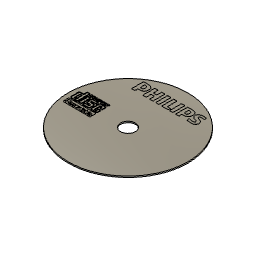
PhillipsCD (Autodesk Fusion 360 design; units mm, degrees)
Autodesk Fusion 360 part; units mm, degrees
(part 1 of 2)
sketch "Sketch1" plane through (0, 0, 0) normal (0, 0, 1) x (1, 0, 0)
  circle A0 centre (0, 0) radius 60
  circle A1 centre (0, 0) radius 7.5
  dimension "d1" = 120
  dimension "d2" = 15
  constraint coincident A0.centre A1.centre
  measures "d1" diameter of A0
  measures "d2" diameter of A1
extrude "Extrude1" add sketch "Sketch1" along normal blind 1.2 makes body 1
sketch "Sketch2" plane through (0, 0, 1.2) normal (0, 0, 1) x (-1, 0, 0)
  circle A0 centre (0, 0) radius 7.5
  circle A1 centre (0, 0) radius 60
  line L0 (-17.284, -38.4124) -> (-15.7727, -38.4124)
  line L1 (-15.7727, -38.4124) -> (-15.7527, -35.3898)
  line L2 (-15.7527, -35.3898) -> (-12.3726, -35.3898)
  line L3 (-12.3726, -35.3898) -> (-12.3726, -47.4806)
  spline S0 degree 3 poles (-12.3726, -47.4806) (-12.3738, -47.4644) (-15.1538, -47.4806) (-16.5283, -47.4806) knots 0 0 0 0 1 1 1 1
  spline S1 degree 3 poles (-16.5283, -47.4806) (-20.0822, -47.4806) (-22.1957, -46.2202) (-22.1957, -42.9463) knots 0 0 0 0 1 1 1 1
  spline S2 degree 3 poles (-22.1957, -42.9463) (-22.1957, -39.9661) (-20.5061, -38.4124) (-17.284, -38.4124) knots 0 0 0 0 1 1 1 1
  spline S3 degree 3 poles (-16.5283, -45.2133) (-16.3508, -45.2133) (-15.9744, -45.2258) (-15.7727, -45.2133) knots 0 0 0 0 1 1 1 1
  line L4 (-15.7727, -45.2133) -> (-15.7727, -40.6798)
  line L5 (-15.7727, -40.6798) -> (-16.5283, -40.6798)
  spline S4 degree 3 poles (-16.5283, -40.6798) (-18.3283, -40.6798) (-18.8516, -41.3599) (-18.8516, -42.8746) knots 0 0 0 0 1 1 1 1
  spline S5 degree 3 poles (-18.8516, -42.8746) (-18.8516, -44.3405) (-18.2346, -45.2133) (-16.5283, -45.2133) knots 0 0 0 0 1 1 1 1
  line L6 (13.6977, -35.3898) -> (13.6977, -40.3019)
  line L7 (13.6977, -40.3019) -> (17.0985, -40.3019)
  line L8 (17.0985, -40.3019) -> (17.0985, -35.3898)
  line L9 (17.0985, -35.3898) -> (20.4985, -35.3898)
  line L10 (20.4985, -35.3898) -> (20.4985, -47.4806)
  line L11 (20.4985, -47.4806) -> (17.0985, -47.4806)
  line L12 (17.0985, -47.4806) -> (17.0985, -42.5685)
  line L13 (17.0985, -42.5685) -> (13.6977, -42.5685)
  line L14 (13.6977, -42.5685) -> (13.6977, -47.4806)
  line L15 (13.6977, -47.4806) -> (10.2969, -47.4806)
  line L16 (10.2969, -47.4806) -> (10.2969, -35.3898)
  line L17 (10.2969, -35.3898) -> (13.6977, -35.3898)
  line L18 (7.6525, -35.3898) -> (7.6525, -47.4806)
  line L19 (7.6525, -47.4806) -> (4.2524, -47.4806)
  line L20 (4.2524, -47.4806) -> (4.2524, -35.3898)
  line L21 (4.2524, -35.3898) -> (7.6525, -35.3898)
  line L22 (-4.7889, -35.3898) -> (1.6076, -35.3898)
  line L23 (1.6076, -35.3898) -> (1.6076, -47.4806)
  line L24 (1.6076, -47.4806) -> (-1.7932, -47.4806)
  line L25 (-1.7932, -47.4806) -> (-1.7932, -37.6572)
  line L26 (-1.7932, -37.6572) -> (-5.1936, -37.6572)
  line L27 (-5.1936, -37.6572) -> (-4.7889, -35.3898)
  line L28 (-6.3271, -35.3898) -> (-6.3271, -47.4806)
  line L29 (-6.3271, -47.4806) -> (-9.7271, -47.4806)
  line L30 (-9.7271, -47.4806) -> (-9.7271, -35.3898)
  line L31 (-9.7271, -35.3898) -> (-6.3271, -35.3898)
  line L32 (-26.73, -44.458) -> (-26.73, -44.0798)
  spline S6 degree 3 poles (-26.73, -44.0798) (-26.73, -42.2239) (-32.3966, -43.0763) (-32.3966, -39.1685) knots 0 0 0 0 1 1 1 1
  spline S7 degree 3 poles (-32.3966, -39.1685) (-32.3966, -36.2373) (-30.3749, -35.3898) (-27.4853, -35.3898) knots 0 0 0 0 1 1 1 1
  spline S8 degree 3 poles (-27.4853, -35.3898) (-26.348, -35.3898) (-24.5129, -35.601) (-23.3292, -35.7677) knots 0 0 0 0 1 1 1 1
  line L33 (-23.3292, -35.7677) -> (-23.3292, -38.4124)
  spline S9 degree 3 poles (-23.3292, -38.4124) (-24.3724, -37.8759) (-26.348, -37.6572) (-27.4853, -37.6572) knots 0 0 0 0 1 1 1 1
  spline S10 degree 3 poles (-27.4853, -37.6572) (-28.7646, -37.6572) (-28.9966, -38.058) (-28.9966, -38.7906) knots 0 0 0 0 1 1 1 1
  spline S11 degree 3 poles (-28.9966, -38.7906) (-28.9966, -40.8725) (-23.3292, -39.9774) (-23.3292, -44.0798) knots 0 0 0 0 1 1 1 1
  spline S12 degree 3 poles (-23.3292, -44.0798) (-23.3292, -46.4616) (-25.6581, -47.4806) (-28.4532, -47.4806) knots 0 0 0 0 1 1 1 1
  spline S13 degree 3 poles (-28.4532, -47.4806) (-30.4338, -47.4806) (-30.741, -47.2978) (-31.6413, -47.1024) knots 0 0 0 0 1 1 1 1
  line L34 (-31.6413, -47.1024) -> (-31.6413, -44.8358)
  spline S14 degree 3 poles (-31.6413, -44.8358) (-30.8351, -45.177) (-29.7091, -45.2133) (-28.6187, -45.2133) knots 0 0 0 0 1 1 1 1
  spline S15 degree 3 poles (-28.6187, -45.2133) (-27.6243, -45.2133) (-26.73, -45.0931) (-26.73, -44.458) knots 0 0 0 0 1 1 1 1
  line L35 (26.9215, -38.4124) -> (28.4332, -38.4124)
  line L36 (28.4332, -38.4124) -> (28.4529, -35.3898)
  line L37 (28.4529, -35.3898) -> (31.8333, -35.3898)
  line L38 (31.8333, -35.3898) -> (31.8333, -47.4806)
  spline S16 degree 3 poles (31.8333, -47.4806) (31.8318, -47.4644) (29.0517, -47.4806) (27.6772, -47.4806) knots 0 0 0 0 1 1 1 1
  spline S17 degree 3 poles (27.6772, -47.4806) (24.1234, -47.4806) (22.0098, -46.2202) (22.0098, -42.9463) knots 0 0 0 0 1 1 1 1
  spline S18 degree 3 poles (22.0098, -42.9463) (22.0098, -39.9661) (23.6995, -38.4124) (26.9215, -38.4124) knots 0 0 0 0 1 1 1 1
  spline S19 degree 3 poles (27.6772, -45.2133) (27.8548, -45.2133) (28.2311, -45.2258) (28.4332, -45.2133) knots 0 0 0 0 1 1 1 1
  line L39 (28.4332, -45.2133) -> (28.4332, -40.6798)
  line L40 (28.4332, -40.6798) -> (27.6772, -40.6798)
  spline S20 degree 3 poles (27.6772, -40.6798) (25.8772, -40.6798) (25.3539, -41.3599) (25.3539, -42.8746) knots 0 0 0 0 1 1 1 1
  spline S21 degree 3 poles (25.3539, -42.8746) (25.3539, -44.3405) (25.9713, -45.2133) (27.6772, -45.2133) knots 0 0 0 0 1 1 1 1
extrude "Extrude2" add sketch "Sketch2" along normal blind 0.0254 separate body contours L0 L1 L2 L3 S0 S1 S2 | L6 L7 L8 L9 L10 L11 L12 L13 L14 L15 L16 L17 | L18 L19 L20 L21 | L22 L23 L24 L25 L26 L27 | L28 L29 L30 L31 | L32 S6 S7 S8 L33 S9 S10 S11 S12 S13 L34 S14 S15 | L35 L36 L37 L38 S16 S17 S18 makes body 2 at (-6.5191, 43.4504, 1.2) makes body 3 at (27.2121, 41.2566, 1.2) makes body 4 at (-0.474, 40.1759, 1.2) makes body 5 at (-11.4305, 41.0575, 1.2) makes body 6 at (13.506, 41.1834, 1.2) makes body 7 at (8.5938, 39.4201, 1.2) makes body 8 at (-30.6999, 41.1834, 1.2)
sketch "Sketch3" plane through (0, 0, 1.2) normal (0, 0, 1) x (-1, 0, 0)
  circle A0 centre (0, 0) radius 7.5
  circle A1 centre (0, 0) radius 60
  spline S0 degree 3 poles (28.7629, 10.1095) (28.3447, 10.1095) (28.0048, 9.7734) (28.0048, 9.3591) knots 0 0 0 0 1 1 1 1
  line L0 (28.0048, 9.3591) -> (28.0048, 4.8183)
  spline S1 degree 3 poles (28.0048, 4.8183) (28.0071, 4.4016) (28.3462, 4.0655) (28.7629, 4.0671) knots 0 0 0 0 1 1 1 1
  line L1 (28.7629, 4.0671) -> (54.5592, 4.0671)
  spline S2 degree 3 poles (54.5592, 4.0671) (54.9759, 4.0648) (55.315, 4.4008) (55.3173, 4.8175) knots 0 0 0 0 1 1 1 1
  line L2 (55.3173, 4.8175) -> (55.3173, 9.3591)
  spline S3 degree 3 poles (55.3173, 9.3591) (55.3173, 9.7734) (54.9789, 10.1095) (54.5592, 10.1095) knots 0 0 0 0 1 1 1 1
  line L3 (54.5592, 10.1095) -> (28.7629, 10.1095)
  spline S4 degree 3 poles (51.7003, -5.31) (52.3594, -5.31) (52.9732, -4.9141) (52.9732, -4.0332) knots 0 0 0 0 1 1 1 1
  spline S5 degree 3 poles (52.9732, -4.0332) (52.9732, -0.3901) (52.9671, -0.1162) (52.9671, 0.5345) knots 0 0 0 0 1 1 1 1
  spline S6 degree 3 poles (52.9671, 0.5345) (52.9671, 0.7869) (52.8021, 1.1521) (52.5819, 1.3386) knots 0 0 0 0 1 1 1 1
  spline S7 degree 3 poles (52.5819, 1.3386) (52.3602, 1.5235) (52.1407, 1.6524) (51.7678, 1.6524) knots 0 0 0 0 1 1 1 1
  spline S8 degree 3 poles (51.7678, 1.6524) (51.3619, 1.6524) (51.134, 1.5312) (50.8808, 1.2972) knots 0 0 0 0 1 1 1 1
  spline S9 degree 3 poles (50.8808, 1.2972) (50.6384, 1.0716) (50.5256, 0.767) (50.5256, 0.4063) knots 0 0 0 0 1 1 1 1
  spline S10 degree 3 poles (50.5256, 0.4063) (50.5256, 0.1646) (50.5355, -3.0357) (50.5355, -4.09) knots 0 0 0 0 1 1 1 1
  spline S11 degree 3 poles (50.5355, -4.09) (50.5355, -4.6402) (50.9744, -5.31) (51.7003, -5.31) knots 0 0 0 0 1 1 1 1
  line L4 (51.1195, -4.0332) -> (51.1195, 0.3802)
  spline S12 degree 3 poles (51.1195, 0.3802) (51.1195, 0.7915) (51.3504, 1.07) (51.7724, 1.07) knots 0 0 0 0 1 1 1 1
  spline S13 degree 3 poles (51.7724, 1.07) (52.1553, 1.0693) (52.3801, 0.7248) (52.3801, 0.4577) knots 0 0 0 0 1 1 1 1
  spline S14 degree 3 poles (52.3801, 0.4577) (52.3801, 0.3764) (52.3901, -2.0076) (52.3901, -4.1) knots 0 0 0 0 1 1 1 1
  spline S15 degree 3 poles (52.3901, -4.1) (52.3901, -4.4744) (52.0809, -4.723) (51.731, -4.723) knots 0 0 0 0 1 1 1 1
  spline S16 degree 3 poles (51.731, -4.723) (51.3811, -4.723) (51.1187, -4.4153) (51.1195, -4.0332) knots 0 0 0 0 1 1 1 1
  spline S17 degree 3 poles (41.3656, -7.4914) (41.1424, -7.4914) (40.8876, -7.4952) (40.6659, -7.4952) knots 0 0 0 0 1 1 1 1
  spline S18 degree 3 poles (40.6659, -7.4952) (40.6659, -8.1283) (40.6697, -9.2708) (40.6659, -9.4457) knots 0 0 0 0 1 1 1 1
  spline S19 degree 3 poles (40.6659, -9.4457) (40.5508, -9.0904) (40.2769, -8.3139) (39.9853, -7.4914) knots 0 0 0 0 1 1 1 1
  spline S20 degree 3 poles (39.9853, -7.4914) (39.7605, -7.4914) (39.5525, -7.4952) (39.3262, -7.4952) knots 0 0 0 0 1 1 1 1
  spline S21 degree 3 poles (39.3262, -7.4952) (39.109, -8.1451) (38.8842, -8.792) (38.6517, -9.4357) knots 0 0 0 0 1 1 1 1
  line L5 (38.6517, -9.4357) -> (38.6517, -7.4952)
  spline S22 degree 3 poles (38.6517, -7.4952) (38.4269, -7.4914) (38.2021, -7.4914) (37.9773, -7.4952) knots 0 0 0 0 1 1 1 1
  line L6 (37.9773, -7.4952) -> (37.975, -10.2061)
  spline S23 degree 3 poles (37.975, -10.2061) (38.3034, -10.2061) (38.6494, -10.2099) (38.9824, -10.2061) knots 0 0 0 0 1 1 1 1
  spline S24 degree 3 poles (38.9824, -10.2061) (39.3346, -9.1442) (39.5019, -8.6684) (39.6615, -8.2357) knots 0 0 0 0 1 1 1 1
  spline S25 degree 3 poles (39.6615, -8.2357) (39.7582, -8.5296) (40.0267, -9.2807) (40.3551, -10.2061) knots 0 0 0 0 1 1 1 1
  line L7 (40.3551, -10.2061) -> (41.3664, -10.2061)
  spline S26 degree 3 poles (41.3664, -10.2061) (41.3702, -9.9513) (41.3641, -8.3139) (41.3656, -7.4914) knots 0 0 0 0 1 1 1 1
  spline S27 degree 3 poles (27.9756, -0.4945) (27.9756, -0.9272) (28.2281, -1.2042) (28.5319, -1.1942) knots 0 0 0 0 1 1 1 1
  spline S28 degree 3 poles (28.5319, -1.1942) (29.0644, -1.1774) (29.9353, -1.2065) (30.5123, -1.1981) knots 0 0 0 0 1 1 1 1
  spline S29 degree 3 poles (30.5123, -1.1981) (30.9405, -1.1935) (31.0156, -0.8006) (31.0156, -0.4108) knots 0 0 0 0 1 1 1 1
  spline S30 degree 3 poles (31.0156, -0.4108) (31.0156, 0.1646) (30.985, 0.2483) (30.985, 0.4539) knots 0 0 0 0 1 1 1 1
  spline S31 degree 3 poles (30.985, 0.4539) (30.985, 0.691) (31.0885, 1.103) (31.4783, 1.103) knots 0 0 0 0 1 1 1 1
  spline S32 degree 3 poles (31.4783, 1.103) (31.8681, 1.103) (32.0246, 0.8184) (32.0246, 0.3818) knots 0 0 0 0 1 1 1 1
  spline S33 degree 3 poles (32.0246, 0.3818) (32.0246, 0.1071) (32.0246, -3.7723) (32.0346, -4.0885) knots 0 0 0 0 1 1 1 1
  spline S34 degree 3 poles (32.0346, -4.0885) (32.0446, -4.3309) (31.8712, -4.6885) (31.5121, -4.6839) knots 0 0 0 0 1 1 1 1
  spline S35 degree 3 poles (31.5121, -4.6839) (31.2397, -4.6854) (31.0179, -4.4667) (31.0164, -4.1944) knots 0 0 0 0 1 1 1 1
  spline S36 degree 3 poles (31.0164, -4.1944) (31.0164, -4.1898) (31.0164, -4.1859) (31.0164, -4.1813) knots 0 0 0 0 1 1 1 1
  spline S37 degree 3 poles (31.0164, -4.1813) (31.0226, -3.7286) (31.0241, -3.5475) (31.0264, -3.0181) knots 0 0 0 0 1 1 1 1
  spline S38 degree 3 poles (31.0264, -3.0181) (31.0287, -2.6153) (30.7693, -2.3582) (30.3987, -2.3582) knots 0 0 0 0 1 1 1 1
  line L8 (30.3987, -2.3582) -> (28.6048, -2.3621)
  spline S39 degree 3 poles (28.6048, -2.3621) (28.1905, -2.3621) (27.9887, -2.6099) (27.9987, -3.0895) knots 0 0 0 0 1 1 1 1
  spline S40 degree 3 poles (27.9987, -3.0895) (28.0086, -3.5728) (28.0048, -3.9166) (28.0048, -5.1189) knots 0 0 0 0 1 1 1 1
  spline S41 degree 3 poles (28.0048, -5.1189) (28.0048, -5.7266) (28.456, -6.8208) (29.6974, -6.8208) knots 0 0 0 0 1 1 1 1
  spline S42 degree 3 poles (29.6974, -6.8208) (30.121, -6.8208) (32.6131, -6.8285) (33.4372, -6.8208) knots 0 0 0 0 1 1 1 1
  spline S43 degree 3 poles (33.4372, -6.8208) (34.1339, -6.8147) (34.6196, -6.3405) (34.8682, -5.8402) knots 0 0 0 0 1 1 1 1
  spline S44 degree 3 poles (34.8682, -5.8402) (35.0884, -5.3975) (35.0316, -5.1397) (35.0316, -4.9333) knots 0 0 0 0 1 1 1 1
  spline S45 degree 3 poles (35.0316, -4.9333) (35.0316, -3.6074) (35.0293, 1.1698) (35.0278, 1.413) knots 0 0 0 0 1 1 1 1
  spline S46 degree 3 poles (35.0278, 1.413) (35.0178, 2.4228) (34.1669, 3.0819) (33.2746, 3.0719) knots 0 0 0 0 1 1 1 1
  spline S47 degree 3 poles (33.2746, 3.0719) (32.1574, 3.0658) (29.9875, 3.0719) (29.547, 3.0719) knots 0 0 0 0 1 1 1 1
  spline S48 degree 3 poles (29.547, 3.0719) (28.6294, 3.0719) (27.9887, 2.1765) (27.9887, 1.535) knots 0 0 0 0 1 1 1 1
  spline S49 degree 3 poles (27.9887, 1.535) (27.991, 0.7716) (27.9764, -0.2152) (27.9756, -0.4945) knots 0 0 0 0 1 1 1 1
  spline S50 degree 3 poles (28.5626, 1.3179) (28.5626, 2.0859) (29.099, 2.5033) (29.501, 2.5033) knots 0 0 0 0 1 1 1 1
  line L9 (29.501, 2.5033) -> (33.3221, 2.5033)
  spline S51 degree 3 poles (33.3221, 2.5033) (34.1869, 2.5033) (34.4593, 1.7637) (34.4593, 1.3447) knots 0 0 0 0 1 1 1 1
  spline S52 degree 3 poles (34.4593, 1.3447) (34.4593, -0.1937) (34.4431, -4.5634) (34.4554, -5.109) knots 0 0 0 0 1 1 1 1
  spline S53 degree 3 poles (34.4554, -5.109) (34.4654, -5.6545) (33.9459, -6.2085) (33.4196, -6.2192) knots 0 0 0 0 1 1 1 1
  spline S54 degree 3 poles (33.4196, -6.2192) (32.894, -6.2292) (30.1486, -6.2192) (29.7473, -6.2085) knots 0 0 0 0 1 1 1 1
  spline S55 degree 3 poles (29.7473, -6.2085) (29.3453, -6.1985) (28.5833, -5.9637) (28.5749, -5.1297) knots 0 0 0 0 1 1 1 1
  spline S56 degree 3 poles (28.5749, -5.1297) (28.5672, -4.2089) (28.5826, -3.5821) (28.5826, -3.3473) knots 0 0 0 0 1 1 1 1
  spline S57 degree 3 poles (28.5826, -3.3473) (28.5826, -3.1125) (28.5826, -2.9253) (28.8818, -2.9352) knots 0 0 0 0 1 1 1 1
  spline S58 degree 3 poles (28.8818, -2.9352) (29.1504, -2.9444) (29.9483, -2.9444) (30.1279, -2.9452) knots 0 0 0 0 1 1 1 1
  spline S59 degree 3 poles (30.1279, -2.9452) (30.279, -2.9475) (30.4486, -2.9966) (30.4402, -3.2859) knots 0 0 0 0 1 1 1 1
  spline S60 degree 3 poles (30.4402, -3.2859) (30.4363, -3.4532) (30.3872, -3.6419) (30.4363, -4.1913) knots 0 0 0 0 1 1 1 1
  spline S61 degree 3 poles (30.4363, -4.1913) (30.4808, -4.7) (30.8054, -5.2808) (31.5075, -5.2632) knots 0 0 0 0 1 1 1 1
  spline S62 degree 3 poles (31.5075, -5.2632) (32.0599, -5.2494) (32.5594, -4.9171) (32.6093, -4.1199) knots 0 0 0 0 1 1 1 1
  spline S63 degree 3 poles (32.6093, -4.1199) (32.6293, -3.8176) (32.607, -0.8029) (32.617, 0.5513) knots 0 0 0 0 1 1 1 1
  spline S64 degree 3 poles (32.617, 0.5513) (32.6185, 1.1751) (32.1205, 1.6854) (31.4975, 1.6984) knots 0 0 0 0 1 1 1 1
  spline S65 degree 3 poles (31.4975, 1.6984) (31.0486, 1.6984) (30.6427, 1.3578) (30.4985, 1.0086) knots 0 0 0 0 1 1 1 1
  spline S66 degree 3 poles (30.4985, 1.0086) (30.3565, 0.6626) (30.4271, -0.2489) (30.4271, -0.2888) knots 0 0 0 0 1 1 1 1
  spline S67 degree 3 poles (30.4271, -0.2888) (30.4271, -0.5068) (30.3435, -0.608) (30.1478, -0.608) knots 0 0 0 0 1 1 1 1
  line L10 (30.1478, -0.608) -> (28.9954, -0.6119)
  spline S68 degree 3 poles (28.9954, -0.6119) (28.8749, -0.6119) (28.5526, -0.6556) (28.5526, -0.2367) knots 0 0 0 0 1 1 1 1
  spline S69 degree 3 poles (28.5526, -0.2367) (28.5526, 0.2391) (28.5649, 0.7984) (28.5626, 1.3179) knots 0 0 0 0 1 1 1 1
  spline S70 degree 3 poles (35.8342, -1.4927) (35.8158, -1.9354) (35.9716, -2.3674) (36.2685, -2.6966) knots 0 0 0 0 1 1 1 1
  spline S71 degree 3 poles (36.2685, -2.6966) (36.5877, -3.0473) (37.0404, -3.2452) (37.5146, -3.2429) knots 0 0 0 0 1 1 1 1
  line L11 (37.5146, -3.2429) -> (39.8625, -3.2429)
  spline S72 degree 3 poles (39.8625, -3.2429) (40.1295, -3.2429) (40.2239, -3.4485) (40.2239, -3.655) knots 0 0 0 0 1 1 1 1
  spline S73 degree 3 poles (40.2239, -3.655) (40.2239, -3.7992) (40.1173, -4.0056) (39.7904, -4.0056) knots 0 0 0 0 1 1 1 1
  line L12 (39.7904, -4.0056) -> (36.6921, -4.0056)
  spline S74 degree 3 poles (36.6921, -4.0056) (36.4197, -4.0179) (36.1979, -4.2289) (36.1718, -4.5005) knots 0 0 0 0 1 1 1 1
  spline S75 degree 3 poles (36.1718, -4.5005) (36.1542, -4.7721) (36.1757, -5.8908) (36.1757, -6.2307) knots 0 0 0 0 1 1 1 1
  spline S76 degree 3 poles (36.1757, -6.2307) (36.178, -6.5584) (36.3875, -6.8216) (36.9744, -6.8108) knots 0 0 0 0 1 1 1 1
  spline S77 degree 3 poles (36.9744, -6.8108) (37.3166, -6.8047) (39.9369, -6.8001) (41.305, -6.8108) knots 0 0 0 0 1 1 1 1
  spline S78 degree 3 poles (41.305, -6.8108) (42.179, -6.8216) (42.9969, -6.0773) (42.9969, -5.2064) knots 0 0 0 0 1 1 1 1
  spline S79 degree 3 poles (42.9969, -5.2064) (42.9992, -4.5534) (42.9931, -2.6989) (42.9931, -2.339) knots 0 0 0 0 1 1 1 1
  spline S80 degree 3 poles (42.9931, -2.339) (42.9931, -1.0623) (42.1575, -0.4546) (41.1907, -0.4546) knots 0 0 0 0 1 1 1 1
  line L13 (41.1907, -0.4546) -> (39.1205, -0.4546)
  spline S81 degree 3 poles (39.1205, -0.4546) (38.6579, -0.4546) (38.6049, -0.2267) (38.6049, -0.0625) knots 0 0 0 0 1 1 1 1
  spline S82 degree 3 poles (38.6049, -0.0625) (38.6049, 0.1017) (38.7584, 0.2981) (39.0047, 0.2981) knots 0 0 0 0 1 1 1 1
  line L14 (39.0047, 0.2981) -> (42.4859, 0.2981)
  spline S83 degree 3 poles (42.4859, 0.2981) (42.7544, 0.2989) (43.003, 0.569) (43.003, 0.8552) knots 0 0 0 0 1 1 1 1
  line L15 (43.003, 0.8552) -> (43.003, 2.4934)
  spline S84 degree 3 poles (43.003, 2.4934) (43.003, 2.9161) (42.5603, 3.0803) (42.3539, 3.0803) knots 0 0 0 0 1 1 1 1
  spline S85 degree 3 poles (42.3539, 3.0803) (42.1475, 3.0803) (38.0509, 3.0681) (37.2131, 3.078) knots 0 0 0 0 1 1 1 1
  spline S86 degree 3 poles (37.2131, 3.078) (36.7366, 3.0842) (36.3115, 2.6798) (36.1872, 2.5056) knots 0 0 0 0 1 1 1 1
  spline S87 degree 3 poles (36.1872, 2.5056) (36.0959, 2.3775) (35.8258, 2.0092) (35.8258, 1.4429) knots 0 0 0 0 1 1 1 1
  spline S88 degree 3 poles (35.8258, 1.4429) (35.8258, 0.2644) (35.8197, -1.9646) (35.8342, -1.4927) knots 0 0 0 0 1 1 1 1
  spline S89 degree 3 poles (36.4235, 1.3486) (36.4235, 2.2762) (37.2499, 2.488) (37.4678, 2.488) knots 0 0 0 0 1 1 1 1
  line L16 (37.4678, 2.488) -> (42.1383, 2.4818)
  spline S90 degree 3 poles (42.1383, 2.4818) (42.4176, 2.4818) (42.4069, 2.2862) (42.4069, 2.0491) knots 0 0 0 0 1 1 1 1
  spline S91 degree 3 poles (42.4069, 2.0491) (42.4069, 1.812) (42.4145, 1.5573) (42.4107, 1.1636) knots 0 0 0 0 1 1 1 1
  spline S92 degree 3 poles (42.4107, 1.1636) (42.4107, 0.9465) (42.2534, 0.8751) (42.0662, 0.8751) knots 0 0 0 0 1 1 1 1
  line L17 (42.0662, 0.8751) -> (38.9563, 0.8751)
  spline S93 degree 3 poles (38.9563, 0.8751) (38.6379, 0.8751) (38.0203, 0.6066) (38.0287, -0.0939) knots 0 0 0 0 1 1 1 1
  spline S94 degree 3 poles (38.0287, -0.0939) (38.0348, -0.4431) (38.3379, -1.0416) (38.9563, -1.0416) knots 0 0 0 0 1 1 1 1
  line L18 (38.9563, -1.0416) -> (41.1815, -1.0416)
  spline S95 degree 3 poles (41.1815, -1.0416) (41.9296, -1.0416) (42.3969, -1.5042) (42.3969, -2.2355) knots 0 0 0 0 1 1 1 1
  spline S96 degree 3 poles (42.3969, -2.2355) (42.3969, -2.9667) (42.393, -4.5005) (42.393, -5.0783) knots 0 0 0 0 1 1 1 1
  spline S97 degree 3 poles (42.393, -5.0783) (42.393, -5.7128) (41.8974, -6.2116) (41.2636, -6.2116) knots 0 0 0 0 1 1 1 1
  line L19 (41.2636, -6.2116) -> (37.0304, -6.2116)
  spline S98 degree 3 poles (37.0304, -6.2116) (36.7389, -6.2108) (36.7427, -5.9768) (36.7427, -5.9116) knots 0 0 0 0 1 1 1 1
  line L20 (36.7427, -5.9116) -> (36.7427, -4.8504)
  spline S99 degree 3 poles (36.7427, -4.8504) (36.7427, -4.6448) (36.7834, -4.5857) (37.042, -4.5926) knots 0 0 0 0 1 1 1 1
  spline S100 degree 3 poles (37.042, -4.5926) (37.401, -4.6026) (39.5157, -4.5887) (39.8372, -4.5887) knots 0 0 0 0 1 1 1 1
  spline S101 degree 3 poles (39.8372, -4.5887) (40.5623, -4.5887) (40.8324, -3.9151) (40.8201, -3.645) knots 0 0 0 0 1 1 1 1
  spline S102 degree 3 poles (40.8201, -3.645) (40.8001, -3.1056) (40.418, -2.6521) (39.7904, -2.6429) knots 0 0 0 0 1 1 1 1
  spline S103 degree 3 poles (39.7904, -2.6429) (39.1627, -2.6321) (38.163, -2.6467) (37.6581, -2.646) knots 0 0 0 0 1 1 1 1
  spline S104 degree 3 poles (37.6581, -2.646) (36.7933, -2.646) (36.422, -2.2232) (36.422, -1.3469) knots 0 0 0 0 1 1 1 1
  line L21 (36.422, -1.3469) -> (36.4243, 1.3501)
  line L22 (36.4243, 1.3501) -> (36.4235, 1.3486)
  spline S105 degree 3 poles (35.1306, -9.4503) (35.1444, -9.6337) (35.1368, -9.8025) (35.2434, -9.946) knots 0 0 0 0 1 1 1 1
  spline S106 degree 3 poles (35.2434, -9.946) (35.3094, -10.0319) (35.3616, -10.1033) (35.5511, -10.1693) knots 0 0 0 0 1 1 1 1
  spline S107 degree 3 poles (35.5511, -10.1693) (35.8588, -10.279) (36.7849, -10.2061) (37.4072, -10.2061) knots 0 0 0 0 1 1 1 1
  spline S108 degree 3 poles (37.4072, -10.2061) (37.4049, -9.3552) (37.411, -7.7293) (37.411, -7.4952) knots 0 0 0 0 1 1 1 1
  spline S109 degree 3 poles (37.411, -7.4952) (37.1908, -7.4952) (36.956, -7.4914) (36.7366, -7.4914) knots 0 0 0 0 1 1 1 1
  spline S110 degree 3 poles (36.7366, -7.4914) (36.7366, -7.6863) (36.7427, -7.9633) (36.7366, -8.1275) knots 0 0 0 0 1 1 1 1
  spline S111 degree 3 poles (36.7366, -8.1275) (36.6391, -8.1206) (36.3207, -8.1229) (36.0775, -8.1283) knots 0 0 0 0 1 1 1 1
  spline S112 degree 3 poles (36.0775, -8.1283) (35.6792, -8.1375) (35.3102, -8.1827) (35.1966, -8.406) knots 0 0 0 0 1 1 1 1
  spline S113 degree 3 poles (35.1966, -8.406) (35.0953, -8.6101) (35.1091, -9.1779) (35.1306, -9.4503) knots 0 0 0 0 1 1 1 1
  spline S114 degree 3 poles (35.8611, -8.8472) (35.9486, -8.7175) (36.465, -8.7636) (36.7358, -8.7643) knots 0 0 0 0 1 1 1 1
  spline S115 degree 3 poles (36.7358, -8.7643) (36.7297, -9.003) (36.7419, -9.3452) (36.7358, -9.5784) knots 0 0 0 0 1 1 1 1
  spline S116 degree 3 poles (36.7358, -9.5784) (36.333, -9.5784) (36.0199, -9.6076) (35.8749, -9.5009) knots 0 0 0 0 1 1 1 1
  spline S117 degree 3 poles (35.8749, -9.5009) (35.7989, -9.4442) (35.7713, -8.9754) (35.8611, -8.8472) knots 0 0 0 0 1 1 1 1
  line L23 (34.2997, -8.0561) -> (33.4042, -8.0561)
  spline S118 degree 3 poles (33.4042, -8.0561) (33.3674, -7.928) (33.2676, -7.5712) (33.2393, -7.4945) knots 0 0 0 0 1 1 1 1
  line L24 (33.2393, -7.4945) -> (32.5648, -7.4945)
  spline S119 degree 3 poles (32.5648, -7.4945) (32.6262, -7.7262) (33.2646, -9.9068) (33.3766, -10.2061) knots 0 0 0 0 1 1 1 1
  spline S120 degree 3 poles (33.3766, -10.2061) (33.5922, -10.2015) (34.1109, -10.2099) (34.3426, -10.2061) knots 0 0 0 0 1 1 1 1
  spline S121 degree 3 poles (34.3426, -10.2061) (34.4746, -9.7833) (35.07, -7.7538) (35.1498, -7.4914) knots 0 0 0 0 1 1 1 1
  line L25 (35.1498, -7.4914) -> (34.4792, -7.4914)
  spline S122 degree 3 poles (34.4792, -7.4914) (34.4117, -7.7185) (34.3411, -7.9226) (34.3004, -8.0554) knots 0 0 0 0 1 1 1 1
  line L26 (34.3004, -8.0554) -> (34.2997, -8.0561)
  spline S123 degree 3 poles (33.8523, -9.5639) (33.751, -9.25) (33.6475, -8.8572) (33.5485, -8.4981) knots 0 0 0 0 1 1 1 1
  line L27 (33.5485, -8.4981) -> (34.1661, -8.4981)
  spline S124 degree 3 poles (34.1661, -8.4981) (34.0664, -8.8411) (33.9383, -9.26) (33.8523, -9.5639) knots 0 0 0 0 1 1 1 1
  spline S125 degree 3 poles (44.5, -6.8239) (44.8507, -6.8239) (45.8313, -6.8139) (46.4942, -6.8131) knots 0 0 0 0 1 1 1 1
  spline S126 degree 3 poles (46.4942, -6.8131) (46.9508, -6.8085) (47.0812, -6.4279) (47.0812, -6.1809) knots 0 0 0 0 1 1 1 1
  line L28 (47.0812, -6.1809) -> (47.0774, 2.3698)
  spline S127 degree 3 poles (47.0774, 2.3698) (47.0774, 2.8425) (46.8019, 3.0773) (46.4328, 3.0773) knots 0 0 0 0 1 1 1 1
  line L29 (46.4328, 3.0773) -> (44.3842, 3.0773)
  spline S128 degree 3 poles (44.3842, 3.0773) (44.0128, 3.0773) (43.8601, 2.6714) (43.8685, 2.3775) knots 0 0 0 0 1 1 1 1
  spline S129 degree 3 poles (43.8685, 2.3775) (43.8747, 2.1719) (43.8785, -2.6061) (43.8785, -6.088) knots 0 0 0 0 1 1 1 1
  spline S130 degree 3 poles (43.8785, -6.088) (43.8785, -6.6282) (44.1701, -6.8231) (44.5008, -6.8231) knots 0 0 0 0 1 1 1 1
  line L30 (44.5008, -6.8231) -> (44.5, -6.8239)
  spline S131 degree 3 poles (44.7241, 2.4811) (44.8369, 2.4811) (45.941, 2.4872) (46.2479, 2.4872) knots 0 0 0 0 1 1 1 1
  spline S132 degree 3 poles (46.2479, 2.4872) (46.4114, 2.4872) (46.5257, 2.409) (46.5257, 2.132) knots 0 0 0 0 1 1 1 1
  spline S133 degree 3 poles (46.5257, 2.132) (46.5257, 1.3908) (46.5134, -5.5095) (46.5134, -5.8601) knots 0 0 0 0 1 1 1 1
  spline S134 degree 3 poles (46.5134, -5.8601) (46.5172, -6.0819) (46.4605, -6.2116) (46.2157, -6.2116) knots 0 0 0 0 1 1 1 1
  line L31 (46.2157, -6.2116) -> (44.7341, -6.2116)
  spline S135 degree 3 poles (44.7341, -6.2116) (44.6113, -6.2116) (44.4525, -6.1341) (44.4525, -5.9077) knots 0 0 0 0 1 1 1 1
  spline S136 degree 3 poles (44.4525, -5.9077) (44.4525, 0.4447) (44.4448, 1.6378) (44.4448, 2.0806) knots 0 0 0 0 1 1 1 1
  spline S137 degree 3 poles (44.4448, 2.0806) (44.4448, 2.5233) (44.6098, 2.4818) (44.7241, 2.4811) knots 0 0 0 0 1 1 1 1
  spline S138 degree 3 poles (32.106, -7.5351) (31.6901, -7.3917) (30.7456, -7.4354) (30.4133, -7.542) knots 0 0 0 0 1 1 1 1
  spline S139 degree 3 poles (30.4133, -7.542) (30.2284, -7.6019) (30.1448, -7.7653) (30.1218, -7.9349) knots 0 0 0 0 1 1 1 1
  spline S140 degree 3 poles (30.1218, -7.9349) (30.0926, -8.1359) (30.0987, -8.2856) (30.0788, -8.4835) knots 0 0 0 0 1 1 1 1
  line L32 (30.0788, -8.4835) -> (30.7632, -8.4835)
  spline S141 degree 3 poles (30.7632, -8.4835) (30.7663, -8.396) (30.7778, -8.1989) (30.8246, -8.1428) knots 0 0 0 0 1 1 1 1
  spline S142 degree 3 poles (30.8246, -8.1428) (30.9305, -8.0193) (31.6786, -8.0362) (31.7561, -8.1636) knots 0 0 0 0 1 1 1 1
  spline S143 degree 3 poles (31.7561, -8.1636) (31.8374, -8.2948) (31.8006, -9.0283) (31.7891, -9.25) knots 0 0 0 0 1 1 1 1
  spline S144 degree 3 poles (31.7891, -9.25) (31.7768, -9.4503) (31.7499, -9.4802) (31.7154, -9.5439) knots 0 0 0 0 1 1 1 1
  spline S145 degree 3 poles (31.7154, -9.5439) (31.6563, -9.6521) (30.8407, -9.6306) (30.8062, -9.5178) knots 0 0 0 0 1 1 1 1
  spline S146 degree 3 poles (30.8062, -9.5178) (30.7693, -9.4043) (30.7693, -9.3367) (30.7693, -9.1825) knots 0 0 0 0 1 1 1 1
  line L33 (30.7693, -9.1825) -> (30.0734, -9.1825)
  spline S147 degree 3 poles (30.0734, -9.1825) (30.0734, -9.4365) (30.0865, -9.6621) (30.1041, -9.8002) knots 0 0 0 0 1 1 1 1
  spline S148 degree 3 poles (30.1041, -9.8002) (30.1248, -9.9721) (30.2921, -10.1186) (30.5453, -10.1762) knots 0 0 0 0 1 1 1 1
  spline S149 degree 3 poles (30.5453, -10.1762) (30.7709, -10.2268) (31.0202, -10.2437) (31.1814, -10.2375) knots 0 0 0 0 1 1 1 1
  spline S150 degree 3 poles (31.1814, -10.2375) (31.3563, -10.2314) (31.6425, -10.2306) (31.8919, -10.1999) knots 0 0 0 0 1 1 1 1
  spline S151 degree 3 poles (31.8919, -10.1999) (32.1328, -10.1693) (32.4359, -10.0802) (32.4612, -9.7818) knots 0 0 0 0 1 1 1 1
  spline S152 degree 3 poles (32.4612, -9.7818) (32.5211, -9.1656) (32.5234, -8.5449) (32.4674, -7.928) knots 0 0 0 0 1 1 1 1
  spline S153 degree 3 poles (32.4674, -7.928) (32.4382, -7.6357) (32.287, -7.5965) (32.106, -7.5336) knots 0 0 0 0 1 1 1 1
  line L34 (32.106, -7.5336) -> (32.106, -7.5351)
  line L35 (29.3015, -7.4937) -> (28.6179, -7.4937)
  line L36 (28.6179, -7.4937) -> (28.6179, -9.4772)
  line L37 (28.6179, -9.4772) -> (27.9833, -9.4772)
  line L38 (27.9833, -9.4772) -> (27.9833, -10.2053)
  line L39 (27.9833, -10.2053) -> (29.9192, -10.2053)
  line L40 (29.9192, -10.2053) -> (29.9192, -9.4718)
  line L41 (29.9192, -9.4718) -> (29.3015, -9.4718)
  line L42 (29.3015, -9.4718) -> (29.3015, -7.4937)
  spline S154 degree 3 poles (47.8861, -9.5792) (47.8861, -9.6398) (47.8861, -10.2069) (48.5038, -10.2069) knots 0 0 0 0 1 1 1 1
  spline S155 degree 3 poles (48.5038, -10.2069) (48.8851, -10.2069) (49.8987, -10.226) (50.6046, -10.2069) knots 0 0 0 0 1 1 1 1
  spline S156 degree 3 poles (50.6046, -10.2069) (50.9077, -10.1769) (51.134, -9.9145) (51.1195, -9.6099) knots 0 0 0 0 1 1 1 1
  spline S157 degree 3 poles (51.1195, -9.6099) (51.1056, -9.2577) (51.1195, -8.8081) (51.1195, -7.0656) knots 0 0 0 0 1 1 1 1
  spline S158 degree 3 poles (51.1195, -7.0656) (51.1172, -6.9136) (51.2261, -6.8231) (51.4133, -6.8231) knots 0 0 0 0 1 1 1 1
  spline S159 degree 3 poles (51.4133, -6.8231) (51.6005, -6.8231) (52.9993, -6.8269) (53.9109, -6.8193) knots 0 0 0 0 1 1 1 1
  spline S160 degree 3 poles (53.9109, -6.8193) (54.7871, -6.8139) (55.503, -5.9469) (55.503, -5.3307) knots 0 0 0 0 1 1 1 1
  spline S161 degree 3 poles (55.503, -5.3307) (55.4953, -2.1449) (55.5068, 0.4493) (55.5068, 1.3685) knots 0 0 0 0 1 1 1 1
  spline S162 degree 3 poles (55.5068, 1.3685) (55.5068, 2.2877) (54.8746, 2.7704) (54.4165, 2.9545) knots 0 0 0 0 1 1 1 1
  spline S163 degree 3 poles (54.4165, 2.9545) (54.1042, 3.0796) (53.66, 3.078) (53.2211, 3.078) knots 0 0 0 0 1 1 1 1
  spline S164 degree 3 poles (53.2211, 3.078) (52.6279, 3.078) (50.0276, 3.0719) (48.6634, 3.078) knots 0 0 0 0 1 1 1 1
  spline S165 degree 3 poles (48.6634, 3.078) (47.8331, 3.0819) (47.8823, 2.465) (47.8823, 2.2662) knots 0 0 0 0 1 1 1 1
  spline S166 degree 3 poles (47.8823, 2.2662) (47.8823, 2.132) (47.8861, -0.3541) (47.8861, -9.5792) knots 0 0 0 0 1 1 1 1
  spline S167 degree 3 poles (48.4876, 2.1366) (48.4876, 2.3737) (48.5552, 2.488) (48.816, 2.4872) knots 0 0 0 0 1 1 1 1
  spline S168 degree 3 poles (48.816, 2.4872) (51.4325, 2.4765) (53.4167, 2.4811) (53.808, 2.4811) knots 0 0 0 0 1 1 1 1
  spline S169 degree 3 poles (53.808, 2.4811) (54.2914, 2.4811) (54.9214, 2.0951) (54.9214, 1.3892) knots 0 0 0 0 1 1 1 1
  spline S170 degree 3 poles (54.9214, 1.3892) (54.9314, -2.0122) (54.9014, -4.8673) (54.9091, -5.2179) knots 0 0 0 0 1 1 1 1
  spline S171 degree 3 poles (54.9091, -5.2179) (54.9214, -5.6929) (54.4035, -6.2238) (53.8633, -6.2223) knots 0 0 0 0 1 1 1 1
  spline S172 degree 3 poles (53.8633, -6.2223) (53.0553, -6.22) (51.7156, -6.2215) (51.1816, -6.2223) knots 0 0 0 0 1 1 1 1
  spline S173 degree 3 poles (51.1816, -6.2223) (50.7795, -6.2223) (50.5309, -6.4195) (50.5386, -6.9067) knots 0 0 0 0 1 1 1 1
  spline S174 degree 3 poles (50.5386, -6.9067) (50.5248, -8.1566) (50.5225, -8.7559) (50.5325, -9.28) knots 0 0 0 0 1 1 1 1
  spline S175 degree 3 poles (50.5325, -9.28) (50.5401, -9.7027) (50.2532, -9.6084) (50.1672, -9.6206) knots 0 0 0 0 1 1 1 1
  spline S176 degree 3 poles (50.1672, -9.6206) (50.178, -9.6199) (49.126, -9.6268) (48.7654, -9.616) knots 0 0 0 0 1 1 1 1
  spline S177 degree 3 poles (48.7654, -9.616) (48.5084, -9.6206) (48.4969, -9.4281) (48.4938, -9.3436) knots 0 0 0 0 1 1 1 1
  spline S178 degree 3 poles (48.4938, -9.3436) (48.4861, -9.1871) (48.4876, 1.9417) (48.4876, 2.1366) knots 0 0 0 0 1 1 1 1
  spline S179 degree 3 poles (42.2204, -7.5106) (41.8122, -7.605) (41.8122, -7.8298) (41.7923, -7.974) knots 0 0 0 0 1 1 1 1
  spline S180 degree 3 poles (41.7923, -7.974) (41.7455, -8.3347) (41.7554, -9.4541) (41.8084, -9.8025) knots 0 0 0 0 1 1 1 1
  spline S181 degree 3 poles (41.8084, -9.8025) (41.8429, -10.0212) (41.9634, -10.0795) (42.1391, -10.1478) knots 0 0 0 0 1 1 1 1
  spline S182 degree 3 poles (42.1391, -10.1478) (42.4483, -10.2713) (43.2854, -10.2805) (43.7404, -10.1685) knots 0 0 0 0 1 1 1 1
  spline S183 degree 3 poles (43.7404, -10.1685) (44.0581, -10.091) (44.0987, -10.0166) (44.157, -9.8025) knots 0 0 0 0 1 1 1 1
  spline S184 degree 3 poles (44.157, -9.8025) (44.2284, -9.5516) (44.2062, -8.3646) (44.1778, -7.9901) knots 0 0 0 0 1 1 1 1
  spline S185 degree 3 poles (44.1778, -7.9901) (44.1532, -7.6518) (43.9307, -7.5689) (43.8256, -7.5367) knots 0 0 0 0 1 1 1 1
  spline S186 degree 3 poles (43.8256, -7.5367) (43.4849, -7.4293) (42.6792, -7.4062) (42.2204, -7.5106) knots 0 0 0 0 1 1 1 1
  spline S187 degree 3 poles (43.3491, -8.0976) (43.4228, -8.1252) (43.4573, -8.1682) (43.4696, -8.2372) knots 0 0 0 0 1 1 1 1
  spline S188 degree 3 poles (43.4696, -8.2372) (43.5041, -8.6308) (43.5102, -9.026) (43.4895, -9.4204) knots 0 0 0 0 1 1 1 1
  spline S189 degree 3 poles (43.4895, -9.4204) (43.4688, -9.5501) (43.4289, -9.5639) (43.3399, -9.5853) knots 0 0 0 0 1 1 1 1
  spline S190 degree 3 poles (43.3399, -9.5853) (43.1327, -9.6368) (42.7322, -9.6291) (42.6018, -9.5861) knots 0 0 0 0 1 1 1 1
  spline S191 degree 3 poles (42.6018, -9.5861) (42.5818, -9.5792) (42.5104, -9.5662) (42.4974, -9.4426) knots 0 0 0 0 1 1 1 1
  spline S192 degree 3 poles (42.4974, -9.4426) (42.4606, -9.1035) (42.4529, -8.4306) (42.4951, -8.2257) knots 0 0 0 0 1 1 1 1
  spline S193 degree 3 poles (42.4951, -8.2257) (42.5158, -8.1206) (42.5665, -8.0953) (42.6393, -8.0861) knots 0 0 0 0 1 1 1 1
  spline S194 degree 3 poles (42.6393, -8.0861) (42.8473, -8.063) (43.2125, -8.0431) (43.3491, -8.0976) knots 0 0 0 0 1 1 1 1
  spline S195 degree 3 poles (46.6208, -7.5451) (46.205, -7.4032) (45.2627, -7.4469) (44.9282, -7.552) knots 0 0 0 0 1 1 1 1
  spline S196 degree 3 poles (44.9282, -7.552) (44.7463, -7.6126) (44.6765, -7.6993) (44.6174, -7.9464) knots 0 0 0 0 1 1 1 1
  spline S197 degree 3 poles (44.6174, -7.9464) (44.5806, -8.1014) (44.5883, -8.2917) (44.5883, -8.4897) knots 0 0 0 0 1 1 1 1
  line L43 (44.5883, -8.4897) -> (45.2742, -8.4897)
  spline S198 degree 3 poles (45.2742, -8.4897) (45.2781, -8.403) (45.2934, -8.2104) (45.3417, -8.1551) knots 0 0 0 0 1 1 1 1
  spline S199 degree 3 poles (45.3417, -8.1551) (45.4453, -8.0316) (46.1957, -8.0477) (46.2732, -8.1751) knots 0 0 0 0 1 1 1 1
  spline S200 degree 3 poles (46.2732, -8.1751) (46.3546, -8.3063) (46.3362, -9.0091) (46.32, -9.2309) knots 0 0 0 0 1 1 1 1
  spline S201 degree 3 poles (46.32, -9.2309) (46.3139, -9.3137) (46.3162, -9.468) (46.2794, -9.5293) knots 0 0 0 0 1 1 1 1
  spline S202 degree 3 poles (46.2794, -9.5293) (46.1996, -9.659) (45.387, -9.6275) (45.321, -9.5293) knots 0 0 0 0 1 1 1 1
  spline S203 degree 3 poles (45.321, -9.5293) (45.2704, -9.4549) (45.2903, -9.339) (45.2742, -9.1902) knots 0 0 0 0 1 1 1 1
  spline S204 degree 3 poles (45.2742, -9.1902) (45.1093, -9.1856) (44.8162, -9.1902) (44.5883, -9.1902) knots 0 0 0 0 1 1 1 1
  spline S205 degree 3 poles (44.5883, -9.1902) (44.5883, -9.4442) (44.6028, -9.6751) (44.619, -9.8132) knots 0 0 0 0 1 1 1 1
  spline S206 degree 3 poles (44.619, -9.8132) (44.6397, -9.9851) (44.8069, -10.1317) (45.0602, -10.1884) knots 0 0 0 0 1 1 1 1
  spline S207 degree 3 poles (45.0602, -10.1884) (45.288, -10.2398) (45.5366, -10.256) (45.6962, -10.2498) knots 0 0 0 0 1 1 1 1
  spline S208 degree 3 poles (45.6962, -10.2498) (45.8727, -10.2452) (46.1589, -10.2429) (46.4067, -10.2107) knots 0 0 0 0 1 1 1 1
  spline S209 degree 3 poles (46.4067, -10.2107) (46.6477, -10.18) (46.9531, -10.091) (46.9776, -9.7917) knots 0 0 0 0 1 1 1 1
  spline S210 degree 3 poles (46.9776, -9.7917) (46.9976, -9.56) (47.0689, -8.7498) (46.9838, -7.938) knots 0 0 0 0 1 1 1 1
  spline S211 degree 3 poles (46.9838, -7.938) (46.9531, -7.6472) (46.8034, -7.6073) (46.6208, -7.5451) knots 0 0 0 0 1 1 1 1
  spline S212 degree 3 poles (46.9584, 6.6436) (46.7866, 6.5807) (46.5986, 6.573) (46.4221, 6.6206) knots 0 0 0 0 1 1 1 1
  spline S213 degree 3 poles (46.4221, 6.6206) (46.2241, 6.6805) (46.1014, 6.8086) (46.0346, 6.9966) knots 0 0 0 0 1 1 1 1
  spline S214 degree 3 poles (46.0346, 6.9966) (46.0147, 7.0534) (46.0139, 7.1071) (46.0016, 7.1677) knots 0 0 0 0 1 1 1 1
  spline S215 degree 3 poles (46.0016, 7.1677) (45.8689, 7.1715) (45.7223, 7.1715) (45.5673, 7.1677) knots 0 0 0 0 1 1 1 1
  spline S216 degree 3 poles (45.5673, 7.1677) (45.6003, 6.8654) (45.6978, 6.6037) (45.875, 6.4441) knots 0 0 0 0 1 1 1 1
  spline S217 degree 3 poles (45.875, 6.4441) (46.0515, 6.2861) (46.3139, 6.1771) (46.683, 6.1894) knots 0 0 0 0 1 1 1 1
  spline S218 degree 3 poles (46.683, 6.1894) (46.9638, 6.1978) (47.2339, 6.3022) (47.4472, 6.4848) knots 0 0 0 0 1 1 1 1
  spline S219 degree 3 poles (47.4472, 6.4848) (47.6513, 6.6636) (47.7733, 6.9436) (47.8347, 7.2697) knots 0 0 0 0 1 1 1 1
  spline S220 degree 3 poles (47.8347, 7.2697) (47.8753, 7.4808) (47.8861, 7.6964) (47.8677, 7.9104) knots 0 0 0 0 1 1 1 1
  spline S221 degree 3 poles (47.8677, 7.9104) (47.8063, 8.5097) (47.4694, 8.9447) (46.8886, 9.046) knots 0 0 0 0 1 1 1 1
  spline S222 degree 3 poles (46.8886, 9.046) (46.6784, 9.0829) (46.3914, 9.0621) (46.218, 8.9892) knots 0 0 0 0 1 1 1 1
  spline S223 degree 3 poles (46.218, 8.9892) (46.0269, 8.9041) (45.8673, 8.7606) (45.763, 8.5795) knots 0 0 0 0 1 1 1 1
  spline S224 degree 3 poles (45.763, 8.5795) (45.6655, 8.4284) (45.598, 8.2672) (45.5796, 8.0332) knots 0 0 0 0 1 1 1 1
  line L44 (45.5796, 8.0332) -> (46.0016, 8.0332)
  spline S225 degree 3 poles (46.0016, 8.0332) (46.0408, 8.1867) (46.0853, 8.3324) (46.1727, 8.4429) knots 0 0 0 0 1 1 1 1
  spline S226 degree 3 poles (46.1727, 8.4429) (46.4098, 8.7483) (46.9561, 8.7383) (47.1971, 8.4429) knots 0 0 0 0 1 1 1 1
  spline S227 degree 3 poles (47.1971, 8.4429) (47.3912, 8.202) (47.4556, 7.658) (47.3666, 7.2467) knots 0 0 0 0 1 1 1 1
  spline S228 degree 3 poles (47.3666, 7.2467) (47.3137, 6.992) (47.1702, 6.7396) (46.9584, 6.6436) knots 0 0 0 0 1 1 1 1
  spline S229 degree 3 poles (48.2659, 6.9413) (48.3296, 6.7549) (48.4477, 6.5585) (48.5843, 6.4411) knots 0 0 0 0 1 1 1 1
  spline S230 degree 3 poles (48.5843, 6.4411) (48.7746, 6.2776) (49.0938, 6.1403) (49.4851, 6.1902) knots 0 0 0 0 1 1 1 1
  spline S231 degree 3 poles (49.4851, 6.1902) (49.8266, 6.2331) (50.1197, 6.3866) (50.2931, 6.5999) knots 0 0 0 0 1 1 1 1
  spline S232 degree 3 poles (50.2931, 6.5999) (50.5969, 6.972) (50.6844, 7.5214) (50.5946, 7.9979) knots 0 0 0 0 1 1 1 1
  spline S233 degree 3 poles (50.5946, 7.9979) (50.4803, 8.6002) (50.122, 8.9731) (49.5588, 9.0261) knots 0 0 0 0 1 1 1 1
  spline S234 degree 3 poles (49.5588, 9.0261) (49.3171, 9.0468) (49.0355, 9.0468) (48.8352, 8.967) knots 0 0 0 0 1 1 1 1
  spline S235 degree 3 poles (48.8352, 8.967) (48.5214, 8.8427) (48.1853, 8.3915) (48.1976, 8.1368) knots 0 0 0 0 1 1 1 1
  line L45 (48.1976, 8.1368) -> (48.6319, 8.1368)
  spline S236 degree 3 poles (48.6319, 8.1368) (48.6503, 8.2304) (48.6887, 8.3194) (48.7447, 8.3977) knots 0 0 0 0 1 1 1 1
  spline S237 degree 3 poles (48.7447, 8.3977) (48.9365, 8.6424) (49.4161, 8.7598) (49.769, 8.581) knots 0 0 0 0 1 1 1 1
  spline S238 degree 3 poles (49.769, 8.581) (49.8995, 8.5143) (50.0299, 8.3432) (50.0782, 8.1936) knots 0 0 0 0 1 1 1 1
  spline S239 degree 3 poles (50.0782, 8.1936) (50.1189, 8.0662) (50.135, 7.9281) (50.135, 7.7608) knots 0 0 0 0 1 1 1 1
  line L46 (50.135, 7.7608) -> (48.1546, 7.7608)
  spline S240 degree 3 poles (48.1546, 7.7608) (48.1546, 7.4462) (48.1876, 7.1777) (48.2674, 6.9406) knots 0 0 0 0 1 1 1 1
  line L47 (48.2674, 6.9406) -> (48.2659, 6.9413)
  spline S241 degree 3 poles (50.1327, 7.3971) (50.1335, 7.2966) (50.1181, 7.1961) (50.0882, 7.1009) knots 0 0 0 0 1 1 1 1
  spline S242 degree 3 poles (50.0882, 7.1009) (50.023, 6.939) (49.9117, 6.8002) (49.7675, 6.702) knots 0 0 0 0 1 1 1 1
  spline S243 degree 3 poles (49.7675, 6.702) (49.6493, 6.6252) (49.512, 6.5823) (49.3716, 6.5777) knots 0 0 0 0 1 1 1 1
  spline S244 degree 3 poles (49.3716, 6.5777) (49.1897, 6.5754) (49.0132, 6.636) (48.8698, 6.748) knots 0 0 0 0 1 1 1 1
  spline S245 degree 3 poles (48.8698, 6.748) (48.7063, 6.8915) (48.6419, 7.1102) (48.6189, 7.3979) knots 0 0 0 0 1 1 1 1
  line L48 (48.6189, 7.3979) -> (50.1327, 7.3971)
  spline S246 degree 3 poles (30.8108, 8.558) (30.9067, 8.4744) (30.9804, 8.3693) (31.0264, 8.2503) knots 0 0 0 0 1 1 1 1
  spline S247 degree 3 poles (31.0264, 8.2503) (31.0732, 8.1184) (31.0832, 7.9734) (31.0832, 7.7946) knots 0 0 0 0 1 1 1 1
  line L49 (31.0832, 7.7946) -> (29.1128, 7.7946)
  spline S248 degree 3 poles (29.1128, 7.7946) (29.1204, 7.5107) (29.1304, 7.3695) (29.1718, 7.1915) knots 0 0 0 0 1 1 1 1
  spline S249 degree 3 poles (29.1718, 7.1915) (29.2294, 6.936) (29.3453, 6.7027) (29.4903, 6.5308) knots 0 0 0 0 1 1 1 1
  spline S250 degree 3 poles (29.4903, 6.5308) (29.6644, 6.3237) (30.0028, 6.1917) (30.411, 6.2247) knots 0 0 0 0 1 1 1 1
  spline S251 degree 3 poles (30.411, 6.2247) (31.1998, 6.2845) (31.5343, 6.9214) (31.575, 7.5851) knots 0 0 0 0 1 1 1 1
  spline S252 degree 3 poles (31.575, 7.5851) (31.6195, 8.2918) (31.2995, 9.0338) (30.4578, 9.0829) knots 0 0 0 0 1 1 1 1
  spline S253 degree 3 poles (30.4578, 9.0829) (30.2376, 9.0967) (29.9913, 9.0806) (29.8202, 9.0153) knots 0 0 0 0 1 1 1 1
  spline S254 degree 3 poles (29.8202, 9.0153) (29.4688, 8.8749) (29.2632, 8.5642) (29.1596, 8.1713) knots 0 0 0 0 1 1 1 1
  line L50 (29.1596, 8.1713) -> (29.6046, 8.1713)
  spline S255 degree 3 poles (29.6046, 8.1713) (29.6982, 8.6516) (30.3819, 8.891) (30.8115, 8.5588) knots 0 0 0 0 1 1 1 1
  line L51 (30.8115, 8.5588) -> (30.8108, 8.558)
  spline S256 degree 3 poles (31.0272, 7.1002) (30.9366, 6.8769) (30.7126, 6.6567) (30.434, 6.6206) knots 0 0 0 0 1 1 1 1
  spline S257 degree 3 poles (30.434, 6.6206) (30.0581, 6.5738) (29.8217, 6.7434) (29.7059, 6.9628) knots 0 0 0 0 1 1 1 1
  spline S258 degree 3 poles (29.7059, 6.9628) (29.6307, 7.1086) (29.5939, 7.2713) (29.5977, 7.4355) knots 0 0 0 0 1 1 1 1
  line L52 (29.5977, 7.4355) -> (31.0847, 7.4355)
  spline S259 degree 3 poles (31.0847, 7.4355) (31.087, 7.3212) (31.0671, 7.2076) (31.0272, 7.1002) knots 0 0 0 0 1 1 1 1
  spline S260 degree 3 poles (51.0335, 8.8312) (51.0972, 8.7967) (51.1049, 8.6002) (51.1133, 8.4215) knots 0 0 0 0 1 1 1 1
  spline S261 degree 3 poles (51.1133, 8.4215) (51.1371, 7.9411) (51.101, 7.414) (51.4087, 7.226) knots 0 0 0 0 1 1 1 1
  spline S262 degree 3 poles (51.4087, 7.226) (51.553, 7.1385) (51.6389, 7.1692) (51.4655, 7.0549) knots 0 0 0 0 1 1 1 1
  spline S263 degree 3 poles (51.4655, 7.0549) (51.2376, 6.9045) (51.1195, 6.6958) (51.078, 6.349) knots 0 0 0 0 1 1 1 1
  spline S264 degree 3 poles (51.078, 6.349) (51.0074, 5.7298) (51.3888, 5.3676) (51.886, 5.2794) knots 0 0 0 0 1 1 1 1
  spline S265 degree 3 poles (51.886, 5.2794) (52.1238, 5.2364) (53.2525, 5.2449) (54.026, 5.2449) knots 0 0 0 0 1 1 1 1
  line L53 (54.026, 5.2449) -> (54.026, 8.9678)
  spline S266 degree 3 poles (54.026, 8.9678) (53.8648, 8.9678) (53.6853, 8.9739) (53.5264, 8.9678) knots 0 0 0 0 1 1 1 1
  line L54 (53.5264, 8.9678) -> (53.5264, 7.3626)
  line L55 (53.5264, 7.3626) -> (52.199, 7.3626)
  spline S267 degree 3 poles (52.199, 7.3626) (52.0532, 7.3565) (51.9113, 7.4102) (51.8062, 7.5107) knots 0 0 0 0 1 1 1 1
  spline S268 degree 3 poles (51.8062, 7.5107) (51.6159, 7.6849) (51.6297, 8.067) (51.6182, 8.4383) knots 0 0 0 0 1 1 1 1
  spline S269 degree 3 poles (51.6182, 8.4383) (51.6113, 8.6163) (51.5875, 8.7944) (51.5468, 8.9678) knots 0 0 0 0 1 1 1 1
  line L56 (51.5468, 8.9678) -> (50.9307, 8.9678)
  spline S270 degree 3 poles (50.9307, 8.9678) (50.9583, 8.8665) (50.9261, 8.8903) (51.0335, 8.8312) knots 0 0 0 0 1 1 1 1
  spline S271 degree 3 poles (51.8185, 6.8278) (51.9527, 6.8984) (52.1024, 6.9337) (52.2543, 6.9314) knots 0 0 0 0 1 1 1 1
  spline S272 degree 3 poles (52.2543, 6.9314) (52.674, 6.9314) (53.2472, 6.9344) (53.5272, 6.9306) knots 0 0 0 0 1 1 1 1
  spline S273 degree 3 poles (53.5272, 6.9306) (53.5272, 6.5155) (53.5311, 6.049) (53.5311, 5.6738) knots 0 0 0 0 1 1 1 1
  spline S274 degree 3 poles (53.5311, 5.6738) (53.2395, 5.6738) (52.6072, 5.6692) (52.2282, 5.6692) knots 0 0 0 0 1 1 1 1
  spline S275 degree 3 poles (52.2282, 5.6692) (51.9934, 5.6699) (51.9343, 5.7091) (51.8185, 5.7758) knots 0 0 0 0 1 1 1 1
  spline S276 degree 3 poles (51.8185, 5.7758) (51.6988, 5.8541) (51.6205, 5.9815) (51.6028, 6.1234) knots 0 0 0 0 1 1 1 1
  spline S277 degree 3 poles (51.6028, 6.1234) (51.5491, 6.4349) (51.6374, 6.7135) (51.8185, 6.8293) knots 0 0 0 0 1 1 1 1
  line L57 (51.8185, 6.8293) -> (51.8185, 6.8278)
  line L58 (41.9357, 6.7012) -> (41.9357, 6.2799)
  line L59 (41.9357, 6.2799) -> (42.3578, 6.2799)
  line L60 (42.3578, 6.2799) -> (42.3578, 8.99)
  line L61 (42.3578, 8.99) -> (41.9296, 8.99)
  spline S278 degree 3 poles (41.9296, 8.99) (41.9296, 8.5534) (41.9235, 8.0808) (41.9235, 7.6457) knots 0 0 0 0 1 1 1 1
  spline S279 degree 3 poles (41.9235, 7.6457) (41.9235, 7.4838) (41.9357, 7.305) (41.8905, 7.1792) knots 0 0 0 0 1 1 1 1
  spline S280 degree 3 poles (41.8905, 7.1792) (41.7524, 6.8002) (41.5053, 6.6667) (41.0465, 6.6667) knots 0 0 0 0 1 1 1 1
  line L62 (41.0465, 6.6667) -> (41.0465, 6.2216)
  spline S281 degree 3 poles (41.0465, 6.2216) (41.0856, 6.2186) (41.1378, 6.1994) (41.183, 6.2009) knots 0 0 0 0 1 1 1 1
  spline S282 degree 3 poles (41.183, 6.2009) (41.5682, 6.207) (41.76, 6.4848) (41.9357, 6.7012) knots 0 0 0 0 1 1 1 1
  spline S283 degree 3 poles (33.9068, 6.2224) (34.1408, 6.1886) (34.3795, 6.2416) (34.5774, 6.372) knots 0 0 0 0 1 1 1 1
  spline S284 degree 3 poles (34.5774, 6.372) (34.6749, 6.438) (34.7562, 6.55) (34.8398, 6.6275) knots 0 0 0 0 1 1 1 1
  line L63 (34.8398, 6.6275) -> (34.8398, 5.2832)
  line L64 (34.8398, 5.2832) -> (35.2918, 5.2855)
  spline S285 degree 3 poles (35.2918, 5.2855) (35.2918, 5.541) (35.2979, 7.6304) (35.2979, 9.0031) knots 0 0 0 0 1 1 1 1
  spline S286 degree 3 poles (35.2979, 9.0031) (35.1736, 9.0031) (35.0355, 9.0054) (34.8644, 9.0031) knots 0 0 0 0 1 1 1 1
  line L65 (34.8644, 9.0031) -> (34.8644, 8.667)
  spline S287 degree 3 poles (34.8644, 8.667) (34.7508, 8.9286) (34.4485, 9.0529) (34.2736, 9.0713) knots 0 0 0 0 1 1 1 1
  spline S288 degree 3 poles (34.2736, 9.0713) (34.0963, 9.089) (33.8032, 9.1343) (33.4763, 8.9064) knots 0 0 0 0 1 1 1 1
  spline S289 degree 3 poles (33.4763, 8.9064) (33.1088, 8.6516) (32.9323, 8.1184) (32.9239, 7.6304) knots 0 0 0 0 1 1 1 1
  spline S290 degree 3 poles (32.9239, 7.6304) (32.9178, 7.2191) (33.0367, 6.8094) (33.2815, 6.5316) knots 0 0 0 0 1 1 1 1
  spline S291 degree 3 poles (33.2815, 6.5316) (33.418, 6.3782) (33.6544, 6.2562) (33.9076, 6.2232) knots 0 0 0 0 1 1 1 1
  line L66 (33.9076, 6.2232) -> (33.9068, 6.2224)
  spline S292 degree 3 poles (34.0112, 8.6954) (34.6212, 8.7767) (34.8836, 8.281) (34.8659, 7.6357) knots 0 0 0 0 1 1 1 1
  spline S293 degree 3 poles (34.8659, 7.6357) (34.8536, 7.1355) (34.6925, 6.6444) (34.1922, 6.6114) knots 0 0 0 0 1 1 1 1
  spline S294 degree 3 poles (34.1922, 6.6114) (33.5761, 6.57) (33.3935, 7.0196) (33.3935, 7.6127) knots 0 0 0 0 1 1 1 1
  spline S295 degree 3 poles (33.3935, 7.6127) (33.3958, 8.2427) (33.6114, 8.6409) (34.0112, 8.6954) knots 0 0 0 0 1 1 1 1
  spline S296 degree 3 poles (44.2246, 6.2009) (45.0295, 6.2608) (45.4085, 7.0365) (45.3517, 7.7654) knots 0 0 0 0 1 1 1 1
  spline S297 degree 3 poles (45.3517, 7.7654) (45.2957, 8.5151) (44.8031, 9.2164) (43.824, 9.0353) knots 0 0 0 0 1 1 1 1
  spline S298 degree 3 poles (43.824, 9.0353) (43.135, 8.9087) (42.7859, 8.1337) (42.8657, 7.4255) knots 0 0 0 0 1 1 1 1
  spline S299 degree 3 poles (42.8657, 7.4255) (42.9371, 6.7518) (43.379, 6.138) (44.2238, 6.2017) knots 0 0 0 0 1 1 1 1
  line L67 (44.2238, 6.2017) -> (44.2246, 6.2009)
  spline S300 degree 3 poles (43.9859, 8.6716) (44.5392, 8.7476) (44.8369, 8.3041) (44.8913, 7.8046) knots 0 0 0 0 1 1 1 1
  spline S301 degree 3 poles (44.8913, 7.8046) (44.952, 7.2529) (44.7103, 6.6344) (44.19, 6.5769) knots 0 0 0 0 1 1 1 1
  spline S302 degree 3 poles (44.19, 6.5769) (43.5931, 6.5078) (43.3092, 7.0656) (43.313, 7.6235) knots 0 0 0 0 1 1 1 1
  spline S303 degree 3 poles (43.313, 7.6235) (43.3169, 8.1168) (43.5471, 8.611) (43.9859, 8.6716) knots 0 0 0 0 1 1 1 1
  spline S304 degree 3 poles (39.0039, 6.6559) (39.1535, 6.4641) (39.363, 6.2539) (39.6584, 6.2124) knots 0 0 0 0 1 1 1 1
  spline S305 degree 3 poles (39.6584, 6.2124) (40.0904, 6.151) (40.4111, 6.2953) (40.6267, 6.5454) knots 0 0 0 0 1 1 1 1
  spline S306 degree 3 poles (40.6267, 6.5454) (40.9513, 6.9245) (41.0426, 7.5698) (40.9045, 8.1015) knots 0 0 0 0 1 1 1 1
  spline S307 degree 3 poles (40.9045, 8.1015) (40.7741, 8.601) (40.4418, 9.0153) (39.93, 9.076) knots 0 0 0 0 1 1 1 1
  spline S308 degree 3 poles (39.93, 9.076) (39.6699, 9.1151) (39.4052, 9.0422) (39.2019, 8.8757) knots 0 0 0 0 1 1 1 1
  spline S309 degree 3 poles (39.2019, 8.8757) (39.1205, 8.8082) (39.0791, 8.7406) (39.0078, 8.6432) knots 0 0 0 0 1 1 1 1
  spline S310 degree 3 poles (39.0078, 8.6432) (39.0078, 8.7583) (39.0039, 8.8903) (39.0055, 8.9916) knots 0 0 0 0 1 1 1 1
  spline S311 degree 3 poles (39.0055, 8.9916) (38.8719, 8.9916) (38.6847, 8.9954) (38.5643, 8.9916) knots 0 0 0 0 1 1 1 1
  line L68 (38.5643, 8.9916) -> (38.5643, 5.2794)
  line L69 (38.5643, 5.2794) -> (39.0093, 5.2794)
  spline S312 degree 3 poles (39.0093, 5.2794) (39.0093, 6.0099) (39.0032, 6.3429) (39.0039, 6.6559) knots 0 0 0 0 1 1 1 1
  spline S313 degree 3 poles (39.6592, 8.6839) (40.4073, 8.7775) (40.5239, 8.0002) (40.4771, 7.3848) knots 0 0 0 0 1 1 1 1
  spline S314 degree 3 poles (40.4771, 7.3848) (40.4625, 7.1715) (40.4196, 6.9789) (40.3175, 6.8493) knots 0 0 0 0 1 1 1 1
  spline S315 degree 3 poles (40.3175, 6.8493) (40.1986, 6.705) (40.026, 6.6152) (39.8395, 6.5991) knots 0 0 0 0 1 1 1 1
  spline S316 degree 3 poles (39.8395, 6.5991) (39.3745, 6.5462) (39.1182, 6.9053) (39.0407, 7.3534) knots 0 0 0 0 1 1 1 1
  spline S317 degree 3 poles (39.0407, 7.3534) (38.9433, 7.9227) (39.0998, 8.611) (39.6584, 8.6831) knots 0 0 0 0 1 1 1 1
  line L70 (39.6584, 8.6831) -> (39.6592, 8.6839)
  spline S318 degree 3 poles (35.9348, 8.5573) (35.9348, 7.9603) (35.9271, 7.5345) (35.9271, 6.9582) knots 0 0 0 0 1 1 1 1
  spline S319 degree 3 poles (35.9271, 6.9582) (35.9271, 6.6828) (36.0644, 6.4633) (36.333, 6.3383) knots 0 0 0 0 1 1 1 1
  spline S320 degree 3 poles (36.333, 6.3383) (36.524, 6.2477) (36.7934, 6.1802) (37.1049, 6.2117) knots 0 0 0 0 1 1 1 1